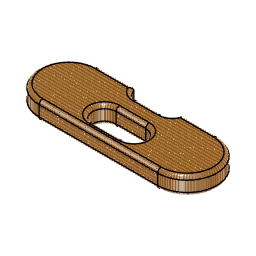
Elastic Clip (Autodesk Fusion 360 design; units mm, degrees)
Autodesk Fusion 360 part; units mm, degrees
sketch "Elastic Clip" plane through (0, 0, 0) normal (0, 0, 1) x (1, 0, 0)
  arc A0 (10, -5) -> (10, 5) centre (10, 0) ccw
  line L0 (-10, -5) -> (10, -5)
  arc A1 (-10, 5) -> (-10, -5) centre (-10, 0) ccw
  line L1 (-2.5, -3.5) -> (0, -3.5)
  arc A2 (-2.5, 0.5) -> (-2.5, -3.5) centre (-2.5, -1.5) ccw
  line L2 (0, 0.5) -> (-2.5, 0.5)
  line L3 (-2.0635, 3.5) -> (2.0635, 3.5)
  arc A3 (-4, 5) -> (-2.0635, 3.5) centre (-2.0635, 5.5) ccw
  arc A4 (2.0635, 3.5) -> (4, 5) centre (2.0635, 5.5) ccw
  line L4 (10, 5) -> (4, 5)
  line L5 (-4, 5) -> (-10, 5)
  line L6 (0, 3.5) -> (0, -5) construction
  line L7 (-15, 0) -> (0, 0) construction
  line L8 (-2.5, -1.5) -> (0, -1.5) construction
  line L9 (0, 0.5) -> (2.5, 0.5)
  arc A5 (2.5, -3.5) -> (2.5, 0.5) centre (2.5, -1.5) ccw
  line L10 (2.5, -3.5) -> (0, -3.5)
  dimension "d1" = 5
  dimension "d2" = 2
  dimension "d3" = 2
  dimension "d4" = 4
  dimension "d5" = 30
  dimension "d6" = 10
  dimension "d8" = 1.5
  dimension "d9" = 1.5
  dimension "d10" = 8
  dimension "d11" = 5
  constraint equal A0 A1
  constraint equal A3 A4
  constraint collinear L4 L5
  constraint midpoint L3 L6.start
  constraint midpoint L0 L6.end
  constraint midpoint A1 L7.start
  constraint coincident L6 L7.end
  constraint perpendicular L6 L7
  constraint coincident A2.centre L8.start
  constraint coincident L6 L8.end
  constraint perpendicular L6 L8
  constraint horizontal L8
  constraint coincident L6 L2.start
  constraint coincident L6 L1.end
  constraint symmetric L1.start L6 A5.start
  constraint symmetric A2.start L6 L9.end
  constraint symmetric A2 L6 A5
  constraint symmetric L6 L1.end L10.end
  constraint tangent L3 A3
  constraint tangent L3 A4
  constraint horizontal L10
  constraint horizontal L3
  constraint horizontal L4
  constraint coincident L7.end origin
  constraint tangent L0 A1
  constraint tangent A0 L0
  measures "d1" distance of A2.centre A5.centre
  measures "d2" radius of A5
  measures "d3" radius of A3
  measures "d4" distance of L1 L2
  measures "d6" distance of L0 L4
  measures "d8" distance of L0 L1
  measures "d9" distance of L3 A3.start
  measures "d10" distance of A3.start A4.end
  measures "d11" radius of A1
extrude "Extrude1" add sketch "Elastic Clip" along normal blind 3
fillet "Fillet1" radius 0.6 2 faces at (-8.15, -0.3516, 3) (-8.15, -0.3516, 0)
named bodies: "Elastic Clip"
